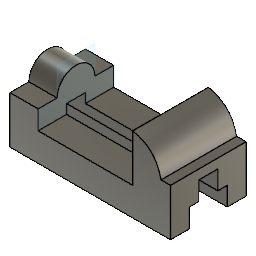
testpart2 v1 (Autodesk Fusion 360 design; units mm, degrees)
Autodesk Fusion 360 part; units mm, degrees
sketch "Sketch1" plane through (0, 0, 0) normal (0, 0, 1) x (1, 0, 0)
  line L0 (17, -8) -> (-17, -8)
  line L1 (-17, -8) -> (-17, 8)
  line L2 (-17, 8) -> (17, 8)
  line L3 (17, 8) -> (17, -8)
  line L4 (17, -8) -> (-17, 8) construction
  line L5 (-17, -8) -> (17, 8) construction
  dimension "d1" = 34
  dimension "d2" = 16
  constraint horizontal L0
  constraint perpendicular L0 L1
  constraint parallel L0 L2
  constraint parallel L1 L3
  constraint coincident L4 origin
  constraint coincident L5 origin
  measures "d1" distance of L1.end L2.end
  measures "d2" distance of L0.end L1.end
extrude "Extrude1" add sketch "Sketch1" along normal blind 16
sketch "Sketch2" plane through (0, 0, 16) normal (0, 0, 1) x (-1, 0, 0)
  line L0 (-17, -8) -> (17, -8)
  line L1 (17, -8) -> (17, 8)
  line L2 (17, 8) -> (-17, 8)
  line L3 (-17, 8) -> (-17, -8)
  line L4 (-17, 8) -> (-15, 8)
  line L5 (-15, 8) -> (-15, -8)
  line L6 (-15, -8) -> (-17, -8)
  line L7 (-17, -8) -> (-17, 8)
  dimension "d5" = 2
  constraint horizontal L4
  constraint vertical L5
  constraint horizontal L6
  constraint vertical L7
  constraint coincident L2.end L3.start
  measures "d5" distance of L2.end L4.end
extrude "Extrude2" cut sketch "Sketch2" against normal blind 6 contours L0 L2 L3 L4 L5 L6 L7
sketch "Sketch3" plane through (0, 8, 0) normal (0, 1, 0) x (-1, 0, 0)
  line L0 (-15, 16) -> (-15, 10)
  line L1 (-15, 10) -> (-17, 10)
  line L2 (-17, 10) -> (-17, 0)
  line L3 (-17, 0) -> (17, 0)
  line L4 (17, 0) -> (17, 16)
  line L5 (17, 16) -> (-15, 16)
  spline S0 degree 5 poles (-15, 10) (-14.9556, 10.1956) (-14.8603, 10.5802) (-14.6976, 11.1373) (-14.4407, 11.8398) (-14.0484, 12.6464) (-13.5785, 13.3749) (-13.0248, 14.0189) (-12.3836, 14.5751) (-11.6585, 15.0467) (-10.8558, 15.4401) (-10.1566, 15.6975) (-9.6022, 15.8603) (-9.2194, 15.9556) (-9.0247, 16) knots 0 0 0 0 0 0 0.1 0.2 0.3 0.4 0.5 0.6 0.7 0.8 0.9 1 1 1 1 1 1
  point P0 (-13, 14)
  constraint coincident L0.end L1.start
  constraint coincident L5 S0.end
extrude "Extrude3" cut sketch "Sketch3" against normal blind 16 contours L0 L5 S0
sketch "Sketch4" plane through (17, 0, 0) normal (1, 0, 0) x (0, 1, 0)
  line L0 (8, 10) -> (-8, 10)
  line L1 (-8, 10) -> (-8, 0)
  line L2 (-8, 0) -> (8, 0)
  line L3 (8, 0) -> (8, 10)
  line L4 (4, 0) -> (-4, 0)
  line L5 (-4, 0) -> (-4, 4)
  line L6 (-4, 4) -> (4, 4)
  line L7 (4, 4) -> (4, 0)
  line L8 (4, 0) -> (-4, 4) construction
  line L9 (-4, 0) -> (4, 4) construction
  point P0 (0, 2)
  dimension "d10" = 8
  dimension "d11" = 4
  constraint horizontal L4
  constraint perpendicular L4 L5
  constraint parallel L4 L6
  constraint parallel L5 L7
  constraint coincident L8 P0
  constraint coincident L9 P0
  measures "d10" distance of L5.end L6.end
  measures "d11" distance of L4.end L5.end
extrude "Extrude4" cut sketch "Sketch4" against normal blind 34 contours L2 L4 L5 L6 L7
sketch "Sketch5" plane through (17, 0, 0) normal (1, 0, 0) x (0, 1, 0)
  line L0 (4, 4) -> (4, 0)
  line L1 (4, 0) -> (8, 0)
  line L2 (8, 0) -> (8, 10)
  line L3 (8, 10) -> (-8, 10)
  line L4 (-8, 10) -> (-8, 0)
  line L5 (-8, 0) -> (-4, 0)
  line L6 (-4, 0) -> (-4, 4)
  line L7 (-4, 4) -> (4, 4)
  line L8 (2, 4) -> (-2, 4)
  line L9 (-2, 4) -> (-2, 8)
  line L10 (-2, 8) -> (2, 8)
  line L11 (2, 8) -> (2, 4)
  line L12 (2, 4) -> (-2, 8) construction
  line L13 (-2, 4) -> (2, 8) construction
  point P0 (0, 6)
  dimension "d14" = 4
  dimension "d15" = 4
  constraint horizontal L8
  constraint perpendicular L8 L9
  constraint parallel L8 L10
  constraint parallel L9 L11
  constraint coincident L12 P0
  constraint coincident L13 P0
  measures "d14" distance of L9.end L10.end
  measures "d15" distance of L8.end L9.end
extrude "Extrude5" cut sketch "Sketch5" against normal blind 34 contours L7 L8 L9 L10 L11
sketch "Sketch6" plane through (0, 0, 16) normal (0, 0, 1) x (-1, 0, 0)
  line L0 (-9.0247, 8) -> (-9.0247, -8)
  line L1 (-9.0247, -8) -> (17, -8)
  line L2 (17, -8) -> (17, 8)
  line L3 (17, 8) -> (-9.0247, 8)
  line L4 (-9, -2) -> (11, -2)
  line L5 (11, -2) -> (11, -8)
  line L6 (11, -8) -> (-9, -8)
  line L7 (-9, -8) -> (-9, -2)
  line L8 (-9, -2) -> (11, -8) construction
  line L9 (11, -2) -> (-9, -8) construction
  point P0 (1, -5)
  dimension "d18" = 20
  dimension "d19" = 6
  constraint horizontal L4
  constraint perpendicular L4 L5
  constraint parallel L4 L6
  constraint parallel L5 L7
  constraint coincident L8 P0
  constraint coincident L9 P0
  measures "d18" distance of L5.end L6.end
  measures "d19" distance of L4.end L5.end
extrude "Extrude6" cut sketch "Sketch6" against normal blind 10 contours L1 L4 L5 L6 L7
sketch "Sketch7" plane through (0, 0, 16) normal (0, 0, 1) x (-1, 0, 0)
  line L0 (-9, -8) -> (-9, -2)
  line L1 (-9, -2) -> (11, -2)
  line L2 (11, -2) -> (11, -8)
  line L3 (11, -8) -> (17, -8)
  line L4 (17, -8) -> (17, 8)
  line L5 (17, 8) -> (-9.0247, 8)
  line L6 (-9.0247, 8) -> (-9.0247, -8)
  line L7 (-9.0247, -8) -> (-9, -8)
  line L8 (11, 2) -> (-9, 2)
  line L9 (-9, 2) -> (-9, 8)
  line L10 (-9, 8) -> (11, 8)
  line L11 (11, 8) -> (11, 2)
  line L12 (11, 2) -> (-9, 8) construction
  line L13 (-9, 2) -> (11, 8) construction
  point P0 (1, 5)
  dimension "d22" = 20
  dimension "d23" = 6
  constraint horizontal L8
  constraint perpendicular L8 L9
  constraint parallel L8 L10
  constraint parallel L9 L11
  constraint coincident L12 P0
  constraint coincident L13 P0
  measures "d22" distance of L9.end L10.end
  measures "d23" distance of L8.end L9.end
extrude "Extrude7" cut sketch "Sketch7" against normal blind 10 contours L5 L8 L9 L10 L11
sketch "Sketch8" plane through (0, 0, 16) normal (0, 0, 1) x (-1, 0, 0)
  line L0 (11, 8) -> (11, 2)
  line L1 (11, 2) -> (-9, 2)
  line L2 (-9, 2) -> (-9, 8)
  line L3 (-9, 8) -> (-9.0247, 8)
  line L4 (-9.0247, 8) -> (-9.0247, -8)
  line L5 (-9.0247, -8) -> (-9, -8)
  line L6 (-9, -8) -> (-9, -2)
  line L7 (-9, -2) -> (11, -2)
  line L8 (11, -2) -> (11, -8)
  line L9 (11, -8) -> (17, -8)
  line L10 (17, -8) -> (17, 8)
  line L11 (17, 8) -> (11, 8)
  line L12 (11, -2) -> (-9, -2)
  line L13 (-9, -2) -> (-9, 2)
  line L14 (-9, 2) -> (11, 2)
  line L15 (11, 2) -> (11, -2)
  line L16 (11, -2) -> (-9, 2) construction
  line L17 (-9, -2) -> (11, 2) construction
  point P0 (1, 0)
  constraint horizontal L12
  constraint perpendicular L12 L13
  constraint parallel L12 L14
  constraint parallel L13 L15
  constraint coincident L16 P0
  constraint coincident L17 P0
  constraint coincident L7.end L8.start
extrude "Extrude8" cut sketch "Sketch8" against normal blind 8 contours L1 L7 L12 L13 L14 L15
sketch "Sketch9" plane through (0, 0, 16) normal (0, 0, 1) x (-1, 0, 0)
  line L0 (11, 8) -> (11, -8)
  line L1 (11, -8) -> (17, -8)
  line L2 (17, -8) -> (17, 8)
  line L3 (17, 8) -> (11, 8)
  line L4 (11, -8) -> (17, -8)
  line L5 (17, -8) -> (17, -4)
  line L6 (17, -4) -> (11, -4)
  line L7 (11, -4) -> (11, -8)
  dimension "d28" = 4
  constraint horizontal L4
  constraint vertical L5
  constraint horizontal L6
  constraint vertical L7
  constraint coincident L0.end L1.start
  measures "d28" distance of L0.end L6.end
extrude "Extrude9" cut sketch "Sketch9" against normal blind 6 contours L0 L1 L2 L4 L5 L6 L7
sketch "Sketch10" plane through (0, 0, 16) normal (0, 0, 1) x (-1, 0, 0)
  line L0 (11, -4) -> (17, -4)
  line L1 (17, -4) -> (17, 8)
  line L2 (17, 8) -> (11, 8)
  line L3 (11, 8) -> (11, -4)
  line L4 (11, 8) -> (17, 8)
  line L5 (17, 8) -> (17, 4)
  line L6 (17, 4) -> (11, 4)
  line L7 (11, 4) -> (11, 8)
  dimension "d31" = 6
  dimension "d32" = 4
  constraint horizontal L4
  constraint vertical L5
  constraint horizontal L6
  constraint vertical L7
  constraint coincident L2.end L3.start
  measures "d31" distance of L2.end L1.end
  measures "d32" distance of L2.end L6.end
extrude "Extrude10" cut sketch "Sketch10" against normal blind 6 contours L1 L2 L3 L4 L5 L6 L7
sketch "Sketch11" plane through (-11, 0, 0) normal (1, 0, 0) x (0, 1, 0)
  line L0 (-4, 16) -> (-4, 10)
  line L1 (-4, 10) -> (-8, 10)
  line L2 (-8, 10) -> (-8, 6)
  line L3 (-8, 6) -> (-2, 6)
  line L4 (-2, 6) -> (-2, 8)
  line L5 (-2, 8) -> (2, 8)
  line L6 (2, 8) -> (2, 6)
  line L7 (2, 6) -> (8, 6)
  line L8 (8, 6) -> (8, 10)
  line L9 (8, 10) -> (4, 10)
  line L10 (4, 10) -> (4, 16)
  line L11 (4, 16) -> (-4, 16)
sketch "Sketch12" plane through (-17, 0, 0) normal (-1, 0, 0) x (0, -1, 0)
  line L0 (4, 10) -> (4, 16)
  line L1 (4, 16) -> (-4, 16)
  line L2 (-4, 16) -> (-4, 10)
  line L3 (-4, 10) -> (-8, 10)
  line L4 (-8, 10) -> (-8, 0)
  line L5 (-8, 0) -> (-4, 0)
  line L6 (-4, 0) -> (-4, 4)
  line L7 (-4, 4) -> (-2, 4)
  line L8 (-2, 4) -> (-2, 8)
  line L9 (-2, 8) -> (2, 8)
  line L10 (2, 8) -> (2, 4)
  line L11 (2, 4) -> (4, 4)
  line L12 (4, 4) -> (4, 0)
  line L13 (4, 0) -> (8, 0)
  line L14 (8, 0) -> (8, 10)
  line L15 (8, 10) -> (4, 10)
  arc A0 (4, 10) -> (-4, 10) centre (0, 10) ccw
  constraint coincident L0.start L15.end
  constraint coincident L2.end L3.start
extrude "Extrude11" cut sketch "Sketch12" against normal blind 6 contours L0 L1 L2 A0
